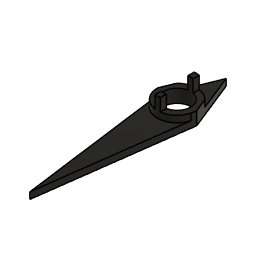
Clock v25 (Autodesk Fusion 360 archive; units mm, degrees)
design "5 lancetta minuti"
Autodesk Fusion 360 part; units mm, degrees
sketch "Schizzo1" plane through (0, 0, 0) normal (0, 0, 1) x (1, 0, 0)
  line L0 (0, -45) -> (6, 0)
  line L1 (6, 0) -> (0, 15)
  line L2 (0, 15) -> (-6, 0)
  line L3 (-6, 0) -> (0, -45)
  line L4 (0, -45) -> (0, 15) construction
  line L5 (6, 0) -> (-6, 0) construction
  circle A0 centre (0, 0) radius 4.15
  circle A1 centre (0, 0) radius 6 construction
  dimension "d1" = 45
  dimension "d2" = 15
  dimension "d3" = 6
  dimension "d12" = 8.3
  dimension "d15" = 12
  constraint vertical L4
  constraint perpendicular L4 L5
  constraint midpoint A0.centre L5
  constraint equal L0 L3
  constraint equal L1 L2
  constraint coincident A0.centre A1.centre
  measures "d1" vertical distance of L0.start L0.end
  measures "d2" vertical distance of L0.end L1.end
  measures "d3" horizontal distance of L0.start L0.end
  measures "d12" diameter of A0
  measures "d15" diameter of A1
extrude "Estrusione1" add sketch "Schizzo1" along normal blind 2
sketch "Schizzo2" plane through (0, 0, 2) normal (0, 0, 1) x (-1, 0, 0)
  line L0 (6, 0) -> (0, 45)
  line L1 (0, 45) -> (-6, 0)
  line L2 (-6, 0) -> (0, -15)
  line L3 (0, -15) -> (6, 0)
  circle A0 centre (0, 0) radius 6
  circle A1 centre (0, 0) radius 4.15
  line L4 (-0.8, 24) -> (0.8, 24)
  line L5 (0.8, 24) -> (0.8, -21)
  line L6 (0.8, -21) -> (-0.8, -21)
  line L7 (-0.8, -21) -> (-0.8, 24)
  circle A2 centre (0, 0) radius 4.15
  circle A3 centre (0, 0) radius 4.15
  line L8 (6, 0) -> (0, 45)
  line L9 (0, 45) -> (-6, 0)
  line L10 (-6, 0) -> (0, -15)
  line L11 (0, -15) -> (6, 0)
  dimension "d6" = 12
  dimension "d7" = 8.3
  dimension "d8" = 0.8
  dimension "d9" = 0.8
  constraint coincident A0.centre A1.centre
  constraint horizontal L4
  constraint vertical L5
  constraint horizontal L6
  constraint vertical L7
  measures "d6" diameter of A0
  measures "d7" diameter of A1
  measures "d8" distance of A0.centre L7
  measures "d9" distance of A0.centre L5
extrude "Estrusione2" add sketch "Schizzo2" along normal blind 5.8 contours A0 A1 L5 L7 A2 A3 | A0 A1 L5 L7 A2 A3
sketch "Schizzo3" plane through (0, 0, 2) normal (0, 0, 1) x (-1, 0, 0)
  line L0 (-0.8, 4.0722) -> (-0.8, 5.9464)
  arc A0 (0.8, 5.9464) -> (-0.8, 5.9464) centre (0, 0) ccw
  line L1 (0.8, 5.9464) -> (0.8, 4.0722)
  arc A1 (0.8, -4.0722) -> (0.8, 4.0722) centre (0, 0) ccw
  line L2 (0.8, -4.0722) -> (0.8, -5.9464)
  arc A2 (-0.8, -5.9464) -> (0.8, -5.9464) centre (0, 0) ccw
  line L3 (-0.8, -5.9464) -> (-0.8, -4.0722)
  arc A3 (-0.8, 4.0722) -> (-0.8, -4.0722) centre (0, 0) ccw
  line L4 (6, 0) -> (0, 45)
  line L5 (0, 45) -> (-6, 0)
  line L6 (-6, 0) -> (0, -15)
  line L7 (0, -15) -> (6, 0)
  circle A4 centre (0, 0) radius 4.15
  circle A5 centre (0, 0) radius 6
  constraint concentric A0 A4
  constraint coincident L3.end A4
  constraint concentric A4 A5
  constraint coincident A2.start A5
extrude "Estrusione3" add sketch "Schizzo3" along normal blind 2 contours L0 L3 A3 L5 L6 A4 A5 | L1 A1 L2 L4 L7 A4 A5

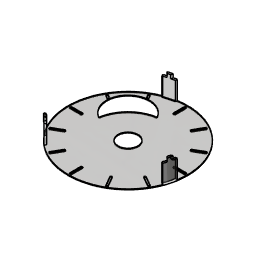
design "10 quadrante"
Autodesk Fusion 360 part; units mm, degrees
sketch "Schizzo1" plane through (0, 0, 0) normal (0, 0, 1) x (1, 0, 0)
  circle A0 centre (0, 0) radius 60
  circle A1 centre (0, 0) radius 10
  circle A2 centre (0, 0) radius 35
  circle A3 centre (-24.0416, 24.0416) radius 21.5
  line L0 (-24.0416, 24.0416) -> (0, 0)
  line L1 (20, 0) -> (2.5, 0)
  dimension "d1" = 120
  dimension "d2" = 20
  dimension "d3" = 70
  dimension "d4" = 43
  dimension "d5" = 135
  dimension "d6" = 34
  constraint coincident A0.centre A1.centre
  constraint concentric A1 A2
  constraint coincident A3.centre L0.start
  measures "d1" diameter of A0
  measures "d2" diameter of A1
  measures "d3" diameter of A2
  measures "d4" diameter of A3
  measures "d5" angle of L0 L1
  measures "d6" distance of A3.centre A0.centre
extrude "Estrusione1" add sketch "Schizzo1" along normal blind 0.8 contours A0 | A2 A3 | A2 A3 picked at (-21.1756, -5.4075) picked at (-19.4046, 19.4046)
sketch "Schizzo2" plane through (0, 0, 0.8) normal (0, 0, 1) x (-1, 0, 0)
  arc A0 (5.3099, -34.5949) -> (34.5949, -5.3099) centre (24.0416, -24.0416) ccw
  arc A1 (5.3099, -34.5949) -> (34.5949, -5.3099) centre (0, 0) ccw
  circle A2 centre (0, 0) radius 10
  circle A3 centre (0, 0) radius 60
  circle A4 centre (0, 0) radius 60
  circle A5 centre (0, 0) radius 58
  circle A6 centre (-57.9555, 15.5291) radius 6
  circle A7 centre (42.4264, 42.4264) radius 6
  circle A8 centre (15.5291, -57.9555) radius 6
  line L0 (15.5291, -57.9555) -> (0, 0) construction
  line L1 (0, 0) -> (-57.9555, 15.5291) construction
  line L2 (0, 0) -> (42.4264, 42.4264) construction
  line L3 (-20, 0) -> (-2.5, 0)
  dimension "d9" = 116
  dimension "d10" = 12
  dimension "d11" = 12
  dimension "d12" = 12
  dimension "d15" = 120
  dimension "d16" = 120
  dimension "d17" = 120
  dimension "d18" = 75
  constraint concentric A1 A4
  constraint concentric A4 A5
  constraint coincident A3 A6.centre
  constraint coincident A4 A7.centre
  constraint coincident A4 A8.centre
  constraint coincident A8.centre L0.start
  constraint coincident A1.centre A2.centre
  constraint coincident A6.centre L1.end
  constraint coincident A7.centre L2.end
  measures "d9" diameter of A5
  measures "d10" diameter of A6
  measures "d11" diameter of A7
  measures "d12" diameter of A8
  measures "d15" angle of L0 L2
  measures "d16" angle of L0 L1
  measures "d17" diameter of A4
  measures "d18" angle of L0 L3
extrude "Estrusione2" add sketch "Schizzo2" along normal blind 18.5 contours A3 A4 A5 A7 | A3 A4 A5 A8 | A3 A4 A5 A6
sketch "Schizzo3" plane through (0, 0, 19.3) normal (0, 0, 1) x (-1, 0, 0)
  arc A0 (9.5764, -57.204) -> (9.6632, -59.2167) centre (15.5291, -57.9555) ccw
  arc A1 (9.6632, -59.2167) -> (21.2398, -56.1148) centre (0, 0) ccw
  arc A2 (21.2398, -56.1148) -> (20.3086, -54.3283) centre (15.5291, -57.9555) ccw
  arc A3 (9.5764, -57.204) -> (20.3086, -54.3283) centre (0, 0) ccw
  circle A4 centre (15.5291, -57.9555) radius 2.5
  dimension "d19" = 5
  constraint concentric A0 A4
  measures "d19" diameter of A4
extrude "Estrusione3" add sketch "Schizzo3" along normal blind 3.5 contours A1 A3 A4
pattern_circular "Serie C1" count 3 over 360 about axis through (0, 0, 1.75) along (0, 0, 1) of "Estrusione3"
sketch "Schizzo4" plane through (0, 0, 0) normal (0, 0, -1) x (1, 0, 0)
  arc A0 (-34.5949, -5.3099) -> (-5.3099, -34.5949) centre (-24.0416, -24.0416) ccw
  arc A1 (-34.5949, -5.3099) -> (-5.3099, -34.5949) centre (0, 0) ccw
  circle A2 centre (0, 0) radius 10
  circle A3 centre (0, 0) radius 60
  line L0 (-58, -0.8) -> (-46, -0.8)
  line L1 (-46, -0.8) -> (-46, 0.8)
  line L2 (-46, 0.8) -> (-58, 0.8)
  line L3 (-58, 0.8) -> (-58, -0.8)
  dimension "d24" = 0.8
  dimension "d25" = 0.8
  dimension "d26" = 58
  dimension "d27" = 12
  constraint horizontal L0
  constraint vertical L1
  constraint horizontal L2
  constraint vertical L3
  measures "d24" distance of A1.centre L0
  measures "d25" distance of A1.centre L2
  measures "d26" distance of A1.centre L3
  measures "d27" distance of L1.end L2.end
extrude "Estrusione4" cut sketch "Schizzo4" against normal blind 0.2 contours L0 L1 L2 L3
pattern_circular "Serie C2" count 12 over 360 about axis through (0, 0, 0) along (0, 0, 1) of "Estrusione4"
sketch "Schizzo5" plane through (0, 0, 0) normal (0, 0, -1) x (1, 0, 0)
  line L0 (0.8, -46) -> (0.8, -58)
  line L1 (0.8, -58) -> (-0.8, -58)
  line L2 (-0.8, -58) -> (-0.8, -46)
  line L3 (-0.8, -46) -> (0.8, -46)
  line L4 (23.6928, -39.4372) -> (29.6928, -49.8295)
  line L5 (29.6928, -49.8295) -> (28.3072, -50.6295)
  line L6 (28.3072, -50.6295) -> (22.3072, -40.2372)
  line L7 (22.3072, -40.2372) -> (23.6928, -39.4372)
  line L8 (40.2372, -22.3072) -> (50.6295, -28.3072)
  line L9 (50.6295, -28.3072) -> (49.8295, -29.6928)
  line L10 (49.8295, -29.6928) -> (39.4372, -23.6928)
  line L11 (39.4372, -23.6928) -> (40.2372, -22.3072)
  line L12 (46, 0.8) -> (58, 0.8)
  line L13 (58, 0.8) -> (58, -0.8)
  line L14 (58, -0.8) -> (46, -0.8)
  line L15 (46, -0.8) -> (46, 0.8)
  line L16 (39.4372, 23.6928) -> (49.8295, 29.6928)
  line L17 (49.8295, 29.6928) -> (50.6295, 28.3072)
  line L18 (50.6295, 28.3072) -> (40.2372, 22.3072)
  line L19 (40.2372, 22.3072) -> (39.4372, 23.6928)
  line L20 (22.3072, 40.2372) -> (28.3072, 50.6295)
  line L21 (28.3072, 50.6295) -> (29.6928, 49.8295)
  line L22 (29.6928, 49.8295) -> (23.6928, 39.4372)
  line L23 (23.6928, 39.4372) -> (22.3072, 40.2372)
  line L24 (-0.8, 46) -> (-0.8, 58)
  line L25 (-0.8, 58) -> (0.8, 58)
  line L26 (0.8, 58) -> (0.8, 46)
  line L27 (0.8, 46) -> (-0.8, 46)
  line L28 (-23.6928, 39.4372) -> (-29.6928, 49.8295)
  line L29 (-29.6928, 49.8295) -> (-28.3072, 50.6295)
  line L30 (-28.3072, 50.6295) -> (-22.3072, 40.2372)
  line L31 (-22.3072, 40.2372) -> (-23.6928, 39.4372)
  line L32 (-40.2372, 22.3072) -> (-50.6295, 28.3072)
  line L33 (-50.6295, 28.3072) -> (-49.8295, 29.6928)
  line L34 (-49.8295, 29.6928) -> (-39.4372, 23.6928)
  line L35 (-39.4372, 23.6928) -> (-40.2372, 22.3072)
  line L36 (-46, -0.8) -> (-58, -0.8)
  line L37 (-58, -0.8) -> (-58, 0.8)
  line L38 (-58, 0.8) -> (-46, 0.8)
  line L39 (-46, 0.8) -> (-46, -0.8)
  line L40 (-45.3242, -27.0917) -> (-49.8295, -29.6928)
  line L41 (-49.8295, -29.6928) -> (-50.6295, -28.3072)
  line L42 (-50.6295, -28.3072) -> (-45.502, -25.3468)
  arc A0 (-34.5949, -5.3099) -> (-45.502, -25.3468) centre (-24.0416, -24.0416) ccw
  arc A1 (-34.5949, -5.3099) -> (-5.3099, -34.5949) centre (0, 0) ccw
  arc A2 (-25.3468, -45.502) -> (-5.3099, -34.5949) centre (-24.0416, -24.0416) ccw
  line L43 (-25.3468, -45.502) -> (-28.3072, -50.6295)
  line L44 (-28.3072, -50.6295) -> (-29.6928, -49.8295)
  line L45 (-29.6928, -49.8295) -> (-27.0917, -45.3242)
  arc A3 (-45.3242, -27.0917) -> (-27.0917, -45.3242) centre (-24.0416, -24.0416) ccw
  circle A4 centre (0, 0) radius 10
  circle A5 centre (0, 0) radius 60
  circle A6 centre (0, 0) radius 35
  circle A7 centre (-24.0416, -24.0416) radius 22.5
  circle A8 centre (-24.0416, -24.0416) radius 21.5
  dimension "d32" = 45
  dimension "d37" = 43
  constraint coincident A1.centre A4.centre
  constraint concentric A3 A7
  constraint concentric A7 A8
  measures "d32" diameter of A7
  measures "d37" diameter of A8
extrude "Estrusione5" add sketch "Schizzo5" along normal up to near side of body 1 contours L40 L42 A7 A8 | L43 L45 A7 A8
sketch "Schizzo7" plane through (0, 0, 0) normal (0, 0, -1) x (1, 0, 0)
  line L0 (-46.2539, -27.6285) -> (-49.8295, -29.6928)
  line L1 (-49.8295, -29.6928) -> (-50.6295, -28.3072)
  line L2 (-50.6295, -28.3072) -> (-46.4645, -25.9026)
  arc A0 (-46.4645, -25.9026) -> (-46.2539, -27.6285) centre (-24.0416, -24.0416) ccw
  line L3 (-25.9026, -46.4645) -> (-28.3072, -50.6295)
  line L4 (-28.3072, -50.6295) -> (-29.6928, -49.8295)
  line L5 (-29.6928, -49.8295) -> (-27.6285, -46.2539)
  arc A1 (-27.6285, -46.2539) -> (-25.9026, -46.4645) centre (-24.0416, -24.0416) ccw
  line L6 (0.8, -46) -> (0.8, -58)
  line L7 (0.8, -58) -> (-0.8, -58)
  line L8 (-0.8, -58) -> (-0.8, -46)
  line L9 (-0.8, -46) -> (0.8, -46)
  line L10 (23.6928, -39.4372) -> (29.6928, -49.8295)
  line L11 (29.6928, -49.8295) -> (28.3072, -50.6295)
  line L12 (28.3072, -50.6295) -> (22.3072, -40.2372)
  line L13 (22.3072, -40.2372) -> (23.6928, -39.4372)
  line L14 (40.2372, -22.3072) -> (50.6295, -28.3072)
  line L15 (50.6295, -28.3072) -> (49.8295, -29.6928)
  line L16 (49.8295, -29.6928) -> (39.4372, -23.6928)
  line L17 (39.4372, -23.6928) -> (40.2372, -22.3072)
  line L18 (46, 0.8) -> (58, 0.8)
  line L19 (58, 0.8) -> (58, -0.8)
  line L20 (58, -0.8) -> (46, -0.8)
  line L21 (46, -0.8) -> (46, 0.8)
  line L22 (39.4372, 23.6928) -> (49.8295, 29.6928)
  line L23 (49.8295, 29.6928) -> (50.6295, 28.3072)
  line L24 (50.6295, 28.3072) -> (40.2372, 22.3072)
  line L25 (40.2372, 22.3072) -> (39.4372, 23.6928)
  line L26 (22.3072, 40.2372) -> (28.3072, 50.6295)
  line L27 (28.3072, 50.6295) -> (29.6928, 49.8295)
  line L28 (29.6928, 49.8295) -> (23.6928, 39.4372)
  line L29 (23.6928, 39.4372) -> (22.3072, 40.2372)
  line L30 (-0.8, 46) -> (-0.8, 58)
  line L31 (-0.8, 58) -> (0.8, 58)
  line L32 (0.8, 58) -> (0.8, 46)
  line L33 (0.8, 46) -> (-0.8, 46)
  line L34 (-23.6928, 39.4372) -> (-29.6928, 49.8295)
  line L35 (-29.6928, 49.8295) -> (-28.3072, 50.6295)
  line L36 (-28.3072, 50.6295) -> (-22.3072, 40.2372)
  line L37 (-22.3072, 40.2372) -> (-23.6928, 39.4372)
  line L38 (-40.2372, 22.3072) -> (-50.6295, 28.3072)
  line L39 (-50.6295, 28.3072) -> (-49.8295, 29.6928)
  line L40 (-49.8295, 29.6928) -> (-39.4372, 23.6928)
  line L41 (-39.4372, 23.6928) -> (-40.2372, 22.3072)
  line L42 (-46, -0.8) -> (-58, -0.8)
  line L43 (-58, -0.8) -> (-58, 0.8)
  line L44 (-58, 0.8) -> (-46, 0.8)
  line L45 (-46, 0.8) -> (-46, -0.8)
  circle A2 centre (0, 0) radius 12.5
  arc A3 (-34.5949, -5.3099) -> (-5.3099, -34.5949) centre (-24.0416, -24.0416) ccw
  arc A4 (-34.5949, -5.3099) -> (-5.3099, -34.5949) centre (0, 0) ccw
  circle A5 centre (0, 0) radius 60
extrude "Estrusione6" cut sketch "Schizzo7" against normal up to surface (0.8 mm away) contours L0 L1 L2 A0 | L3 L4 L5 A1 | L6 L7 L8 L9 | L10 L11 L12 L13 | L14 L15 L16 L17 | L18 L19 L20 L21 | L22 L23 L24 L25 | L26 L27 L28 L29 | L30 L31 L32 L33 | L34 L35 L36 L37 | L38 L39 L40 L41 | L42 L43 L44 L45

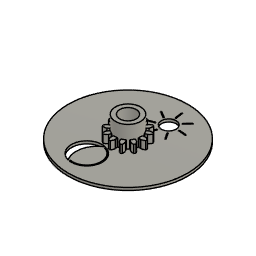
design "9 night and day"
description: Spur Gear; Module: 1.000000; Num Teeth: 12; Pressure Angle: 20.000000; Backlash: 0.00 mm
Autodesk Fusion 360 part; units mm, degrees
sketch "Schizzo1" plane through (0, 0, 0) normal (0, 0, 1) x (1, 0, 0)
  circle A0 centre (0, 0) radius 22.5
  dimension "d1" = 45
  constraint coincident A0.centre origin
  measures "d1" diameter of A0
extrude "Estrusione1" add sketch "Schizzo1" along normal blind 1 makes body 1
sketch "Schizzo1 (2)" plane through (0, 0, 0) normal (0, 0, 1) x (1, 0, 0) in component "Spur Gear (12 teeth)"
  circle A0 centre (0, 0) radius 4.7492
extrude "Estrusione1'" add sketch "Schizzo1 (2)" along normal blind 5 separate body makes body 2 in component "Spur Gear (12 teeth)"
sketch "Schizzo2" plane through (0, 0, 0) normal (0, 0, 1) x (1, 0, 0) in component "Spur Gear (12 teeth)"
  spline S0 degree 5 poles (5.5783, -0.8192) (5.5823, -0.8197) (5.5902, -0.8208) (5.6021, -0.8219) (5.6181, -0.8228) (5.6381, -0.8229) (5.6583, -0.8223) (5.6784, -0.8212) (5.6986, -0.8199) (5.7188, -0.8184) (5.7391, -0.8168) (5.7593, -0.8149) (5.7796, -0.8127) (5.7999, -0.8102) (5.8203, -0.8073) (5.8406, -0.8041) (5.861, -0.8006) (5.8814, -0.7969) (5.9018, -0.793) (5.9222, -0.7888) (5.9426, -0.7845) (5.9631, -0.7799) (5.9835, -0.7752) (6.0039, -0.7702) (6.0244, -0.765) (6.0448, -0.7596) (6.0653, -0.7539) (6.0857, -0.7481) (6.1061, -0.7421) (6.1266, -0.7359) (6.147, -0.7295) (6.1675, -0.7229) (6.1879, -0.7161) (6.2083, -0.7092) (6.2288, -0.7021) (6.2492, -0.6947) (6.2696, -0.6873) (6.29, -0.6796) (6.3104, -0.6717) (6.3308, -0.6637) (6.3512, -0.6555) (6.3715, -0.6472) (6.3919, -0.6387) (6.4122, -0.63) (6.4325, -0.6211) (6.4528, -0.6121) (6.4731, -0.6029) (6.4934, -0.5936) (6.5137, -0.5841) (6.5339, -0.5744) (6.5541, -0.5646) (6.5743, -0.5546) (6.5945, -0.5445) (6.6147, -0.5342) (6.6348, -0.5238) (6.655, -0.5132) (6.6751, -0.5024) (6.6951, -0.4915) (6.7152, -0.4805) (6.7352, -0.4693) (6.7552, -0.4579) (6.7752, -0.4464) (6.7952, -0.4348) (6.8151, -0.423) (6.835, -0.4111) (6.8549, -0.399) (6.8747, -0.3867) (6.8945, -0.3744) (6.9143, -0.3619) (6.9341, -0.3492) (6.9538, -0.3364) (6.9695, -0.3261) (6.9813, -0.3182) (6.9892, -0.313) (6.9931, -0.3103) knots 0 0 0 0 0 0 0.01428571 0.02857143 0.04285714 0.05714286 0.07142857 0.08571429 0.1 0.11428571 0.12857143 0.14285714 0.15714286 0.17142857 0.18571429 0.2 0.21428571 0.22857143 0.24285714 0.25714286 0.27142857 0.28571429 0.3 0.31428571 0.32857143 0.34285714 0.35714286 0.37142857 0.38571429 0.4 0.41428571 0.42857143 0.44285714 0.45714286 0.47142857 0.48571429 0.5 0.51428571 0.52857143 0.54285714 0.55714286 0.57142857 0.58571429 0.6 0.61428571 0.62857143 0.64285714 0.65714286 0.67142857 0.68571429 0.7 0.71428571 0.72857143 0.74285714 0.75714286 0.77142857 0.78571429 0.8 0.81428571 0.82857143 0.84285714 0.85714286 0.87142857 0.88571429 0.9 0.91428571 0.92857143 0.94285714 0.95714286 0.97142857 0.98571429 1 1 1 1 1 1
  spline S1 degree 5 poles (5.5783, 0.8192) (5.5823, 0.8197) (5.5902, 0.8208) (5.6021, 0.8219) (5.6181, 0.8228) (5.6381, 0.8229) (5.6583, 0.8223) (5.6784, 0.8212) (5.6986, 0.8199) (5.7188, 0.8184) (5.7391, 0.8168) (5.7593, 0.8149) (5.7796, 0.8127) (5.7999, 0.8102) (5.8203, 0.8073) (5.8406, 0.8041) (5.861, 0.8006) (5.8814, 0.7969) (5.9018, 0.793) (5.9222, 0.7888) (5.9426, 0.7845) (5.9631, 0.7799) (5.9835, 0.7752) (6.0039, 0.7702) (6.0244, 0.765) (6.0448, 0.7596) (6.0653, 0.7539) (6.0857, 0.7481) (6.1061, 0.7421) (6.1266, 0.7359) (6.147, 0.7295) (6.1675, 0.7229) (6.1879, 0.7161) (6.2083, 0.7092) (6.2288, 0.7021) (6.2492, 0.6947) (6.2696, 0.6873) (6.29, 0.6796) (6.3104, 0.6717) (6.3308, 0.6637) (6.3512, 0.6555) (6.3715, 0.6472) (6.3919, 0.6387) (6.4122, 0.63) (6.4325, 0.6211) (6.4528, 0.6121) (6.4731, 0.6029) (6.4934, 0.5936) (6.5137, 0.5841) (6.5339, 0.5744) (6.5541, 0.5646) (6.5743, 0.5546) (6.5945, 0.5445) (6.6147, 0.5342) (6.6348, 0.5238) (6.655, 0.5132) (6.6751, 0.5024) (6.6951, 0.4915) (6.7152, 0.4805) (6.7352, 0.4693) (6.7552, 0.4579) (6.7752, 0.4464) (6.7952, 0.4348) (6.8151, 0.423) (6.835, 0.4111) (6.8549, 0.399) (6.8747, 0.3867) (6.8945, 0.3744) (6.9143, 0.3619) (6.9341, 0.3492) (6.9538, 0.3364) (6.9695, 0.3261) (6.9813, 0.3182) (6.9892, 0.313) (6.9931, 0.3103) knots 0 0 0 0 0 0 0.01428571 0.02857143 0.04285714 0.05714286 0.07142857 0.08571429 0.1 0.11428571 0.12857143 0.14285714 0.15714286 0.17142857 0.18571429 0.2 0.21428571 0.22857143 0.24285714 0.25714286 0.27142857 0.28571429 0.3 0.31428571 0.32857143 0.34285714 0.35714286 0.37142857 0.38571429 0.4 0.41428571 0.42857143 0.44285714 0.45714286 0.47142857 0.48571429 0.5 0.51428571 0.52857143 0.54285714 0.55714286 0.57142857 0.58571429 0.6 0.61428571 0.62857143 0.64285714 0.65714286 0.67142857 0.68571429 0.7 0.71428571 0.72857143 0.74285714 0.75714286 0.77142857 0.78571429 0.8 0.81428571 0.82857143 0.84285714 0.85714286 0.87142857 0.88571429 0.9 0.91428571 0.92857143 0.94285714 0.95714286 0.97142857 0.98571429 1 1 1 1 1 1
  arc A0 (6.9931, -0.3103) -> (6.9931, 0.3103) centre (0, 0) ccw
  line L0 (4.6889, -0.69) -> (5.5783, -0.8192)
  line L1 (4.6889, 0.69) -> (5.5783, 0.8192)
  line L2 (4.6889, -0.69) -> (4.6889, 0.69)
  point P0 (5.6763, -0.8213)
  point P1 (5.7758, -0.8131)
  point P2 (5.8761, -0.7978)
  point P3 (5.977, -0.7767)
  point P4 (6.0784, -0.7502)
  point P5 (6.1802, -0.7187)
  point P6 (6.2821, -0.6825)
  point P7 (6.3842, -0.6419)
  point P8 (6.4862, -0.5969)
  point P9 (6.5882, -0.5477)
  point P10 (6.6899, -0.4943)
  point P11 (6.7914, -0.437)
  point P12 (6.8925, -0.3756)
  point P13 (5.6763, 0.8213)
  point P14 (5.7758, 0.8131)
  point P15 (5.8761, 0.7978)
  point P16 (5.977, 0.7767)
  point P17 (6.0784, 0.7502)
  point P18 (6.1802, 0.7187)
  point P19 (6.2821, 0.6825)
  point P20 (6.3842, 0.6419)
  point P21 (6.4862, 0.5969)
  point P22 (6.5882, 0.5477)
  point P23 (6.6899, 0.4943)
  point P24 (6.7914, 0.437)
  point P25 (6.8925, 0.3756)
extrude "Estrusione2" add sketch "Schizzo2" along normal blind 5 bodies 2 in component "Spur Gear (12 teeth)"
fillet "Raccordo1" radius 0.1 2 edges at (4.6986, -0.6914, 2.5) (4.6986, 0.6914, 2.5) on bodies 2 in component "Spur Gear (12 teeth)"
pattern_circular "Serie C1" count 12 over 360 about axis through (0, 0, 0) along (0, 0, 1) of "Estrusione2", "Raccordo1" in component "Spur Gear (12 teeth)"
sketch "Schizzo3" plane through (0, 0, 0) normal (0, 0, 1) x (1, 0, 0) in component "Spur Gear (12 teeth)"
  circle A0 centre (0, 0) radius 6 construction
combine "Combina1" operation add target body 1 tool bodies 2
extrude "Estrusione2'" cut 1 faces at (0.3611, -1.5413, 5) along direction (0, 0, -1) blind 1 on bodies 1 bodies 1
sketch "Schizzo2 (2)" plane through (0, 0, 4) normal (0, 0, 1) x (-1, 0, 0)
  arc A0 (-4.4499, 1.6593) -> (-4.6834, 0.788) centre (0, 0) ccw
  arc A1 (-4.7964, 0.7056) -> (-4.6834, 0.788) centre (-4.782, 0.8046) ccw
  line L0 (-4.7964, 0.7056) -> (-5.5783, 0.8192)
  spline S0 degree 3 poles (-6.9931, 0.3103) (-6.7925, 0.4447) (-6.5771, 0.5635) (-6.0115, 0.7938) (-5.7809, 0.814) (-5.6435, 0.8238) (-5.6102, 0.8238) (-5.5783, 0.8192) knots -0.02978 -0.02978 -0.02978 -0.02978 -0.021848 -0.021848 -0.009668 -0.009668 0 0 0 0
  arc A2 (-6.9931, 0.3103) -> (-6.9931, -0.3103) centre (0, 0) ccw
  spline S1 degree 3 poles (-5.5783, -0.8192) (-5.6911, -0.8355) (-5.8671, -0.8005) (-6.0076, -0.7707) (-6.1286, -0.7409) (-6.536, -0.586) (-6.7735, -0.4574) (-6.9931, -0.3103) knots -0.176502 -0.176502 -0.176502 -0.176502 -0.131302 -0.131302 -0.079288 -0.079288 0 0 0 0
  line L1 (-5.5783, -0.8192) -> (-4.7964, -0.7056)
  arc A3 (-4.6834, -0.788) -> (-4.7964, -0.7056) centre (-4.782, -0.8046) ccw
  arc A4 (-4.6834, -0.788) -> (-4.4499, -1.6593) centre (0, 0) ccw
  arc A5 (-4.5066, -1.7871) -> (-4.4499, -1.6593) centre (-4.5436, -1.6942) ccw
  line L2 (-4.5066, -1.7871) -> (-5.2406, -2.0798)
  spline S2 degree 3 poles (-6.2114, -3.2278) (-6.1048, -3.0111) (-5.9777, -2.8005) (-5.603, -2.3183) (-5.4134, -2.1855) (-5.2993, -2.1084) (-5.2705, -2.0917) (-5.2406, -2.0798) knots -0.02978 -0.02978 -0.02978 -0.02978 -0.021848 -0.021848 -0.009668 -0.009668 0 0 0 0
  arc A6 (-6.2114, -3.2278) -> (-5.901, -3.7653) centre (0, 0) ccw
  spline S3 degree 3 poles (-4.4214, -3.4986) (-4.5109, -3.5691) (-4.6808, -3.6268) (-4.8174, -3.6712) (-4.9371, -3.7059) (-5.3674, -3.7755) (-5.6373, -3.7829) (-5.901, -3.7653) knots -0.176502 -0.176502 -0.176502 -0.176502 -0.131302 -0.131302 -0.079288 -0.079288 0 0 0 0
  line L3 (-4.4214, -3.4986) -> (-3.801, -3.0093)
  arc A7 (-3.6619, -3.0241) -> (-3.801, -3.0093) centre (-3.739, -3.0878) ccw
  arc A8 (-3.6619, -3.0241) -> (-3.0241, -3.6619) centre (0, 0) ccw
  arc A9 (-3.0093, -3.801) -> (-3.0241, -3.6619) centre (-3.0878, -3.739) ccw
  line L4 (-3.0093, -3.801) -> (-3.4986, -4.4214)
  spline S4 degree 3 poles (-3.7653, -5.901) (-3.7814, -5.6601) (-3.7766, -5.4142) (-3.6932, -4.8092) (-3.5954, -4.5994) (-3.5352, -4.4756) (-3.5185, -4.4467) (-3.4986, -4.4214) knots -0.02978 -0.02978 -0.02978 -0.02978 -0.021848 -0.021848 -0.009668 -0.009668 0 0 0 0
  arc A10 (-3.7653, -5.901) -> (-3.2278, -6.2114) centre (0, 0) ccw
  spline S5 degree 3 poles (-2.0798, -5.2406) (-2.122, -5.3464) (-2.2403, -5.4813) (-2.3364, -5.5881) (-2.4227, -5.678) (-2.7605, -5.9534) (-2.9906, -6.0947) (-3.2278, -6.2114) knots -0.176502 -0.176502 -0.176502 -0.176502 -0.131302 -0.131302 -0.079288 -0.079288 0 0 0 0
  line L5 (-2.0798, -5.2406) -> (-1.7871, -4.5066)
  arc A11 (-1.6593, -4.4499) -> (-1.7871, -4.5066) centre (-1.6942, -4.5436) ccw
  arc A12 (-1.6593, -4.4499) -> (-0.788, -4.6834) centre (0, 0) ccw
  arc A13 (-0.7056, -4.7964) -> (-0.788, -4.6834) centre (-0.8046, -4.782) ccw
  line L6 (-0.7056, -4.7964) -> (-0.8192, -5.5783)
  spline S6 degree 3 poles (-0.3103, -6.9931) (-0.4447, -6.7925) (-0.5635, -6.5771) (-0.7938, -6.0115) (-0.814, -5.7809) (-0.8238, -5.6435) (-0.8238, -5.6102) (-0.8192, -5.5783) knots -0.02978 -0.02978 -0.02978 -0.02978 -0.021848 -0.021848 -0.009668 -0.009668 0 0 0 0
  arc A14 (-0.3103, -6.9931) -> (0.3103, -6.9931) centre (0, 0) ccw
  spline S7 degree 3 poles (0.8192, -5.5783) (0.8355, -5.6911) (0.8005, -5.8671) (0.7707, -6.0076) (0.7409, -6.1286) (0.586, -6.536) (0.4574, -6.7735) (0.3103, -6.9931) knots -0.176502 -0.176502 -0.176502 -0.176502 -0.131302 -0.131302 -0.079288 -0.079288 0 0 0 0
  line L7 (0.8192, -5.5783) -> (0.7056, -4.7964)
  arc A15 (0.788, -4.6834) -> (0.7056, -4.7964) centre (0.8046, -4.782) ccw
  arc A16 (0.788, -4.6834) -> (1.6593, -4.4499) centre (0, 0) ccw
  arc A17 (1.7871, -4.5066) -> (1.6593, -4.4499) centre (1.6942, -4.5436) ccw
  line L8 (1.7871, -4.5066) -> (2.0798, -5.2406)
  spline S8 degree 3 poles (3.2278, -6.2114) (3.0111, -6.1048) (2.8005, -5.9777) (2.3183, -5.603) (2.1855, -5.4134) (2.1084, -5.2993) (2.0917, -5.2705) (2.0798, -5.2406) knots -0.02978 -0.02978 -0.02978 -0.02978 -0.021848 -0.021848 -0.009668 -0.009668 0 0 0 0
  arc A18 (3.2278, -6.2114) -> (3.7653, -5.901) centre (0, 0) ccw
  spline S9 degree 3 poles (3.4986, -4.4214) (3.5691, -4.5109) (3.6268, -4.6808) (3.6712, -4.8174) (3.7059, -4.9371) (3.7755, -5.3674) (3.7829, -5.6373) (3.7653, -5.901) knots -0.176502 -0.176502 -0.176502 -0.176502 -0.131302 -0.131302 -0.079288 -0.079288 0 0 0 0
  line L9 (3.4986, -4.4214) -> (3.0093, -3.801)
  arc A19 (3.0241, -3.6619) -> (3.0093, -3.801) centre (3.0878, -3.739) ccw
  arc A20 (3.0241, -3.6619) -> (3.6619, -3.0241) centre (0, 0) ccw
  arc A21 (3.801, -3.0093) -> (3.6619, -3.0241) centre (3.739, -3.0878) ccw
  line L10 (3.801, -3.0093) -> (4.4214, -3.4986)
  spline S10 degree 3 poles (5.901, -3.7653) (5.6601, -3.7814) (5.4142, -3.7766) (4.8092, -3.6932) (4.5994, -3.5954) (4.4756, -3.5352) (4.4467, -3.5185) (4.4214, -3.4986) knots -0.02978 -0.02978 -0.02978 -0.02978 -0.021848 -0.021848 -0.009668 -0.009668 0 0 0 0
  arc A22 (5.901, -3.7653) -> (6.2114, -3.2278) centre (0, 0) ccw
  spline S11 degree 3 poles (5.2406, -2.0798) (5.3464, -2.122) (5.4813, -2.2403) (5.5881, -2.3364) (5.678, -2.4227) (5.9534, -2.7605) (6.0947, -2.9906) (6.2114, -3.2278) knots -0.176502 -0.176502 -0.176502 -0.176502 -0.131302 -0.131302 -0.079288 -0.079288 0 0 0 0
  line L11 (5.2406, -2.0798) -> (4.5066, -1.7871)
  arc A23 (4.4499, -1.6593) -> (4.5066, -1.7871) centre (4.5436, -1.6942) ccw
  arc A24 (4.4499, -1.6593) -> (4.6834, -0.788) centre (0, 0) ccw
  arc A25 (4.7964, -0.7056) -> (4.6834, -0.788) centre (4.782, -0.8046) ccw
  line L12 (4.7964, -0.7056) -> (5.5783, -0.8192)
  spline S12 degree 3 poles (6.9931, -0.3103) (6.7925, -0.4447) (6.5771, -0.5635) (6.0115, -0.7938) (5.7809, -0.814) (5.6435, -0.8238) (5.6102, -0.8238) (5.5783, -0.8192) knots -0.02978 -0.02978 -0.02978 -0.02978 -0.021848 -0.021848 -0.009668 -0.009668 0 0 0 0
  arc A26 (6.9931, -0.3103) -> (6.9931, 0.3103) centre (0, 0) ccw
  spline S13 degree 3 poles (5.5783, 0.8192) (5.6911, 0.8355) (5.8671, 0.8005) (6.0076, 0.7707) (6.1286, 0.7409) (6.536, 0.586) (6.7735, 0.4574) (6.9931, 0.3103) knots -0.176502 -0.176502 -0.176502 -0.176502 -0.131302 -0.131302 -0.079288 -0.079288 0 0 0 0
  line L13 (5.5783, 0.8192) -> (4.7964, 0.7056)
  arc A27 (4.6834, 0.788) -> (4.7964, 0.7056) centre (4.782, 0.8046) ccw
  arc A28 (4.6834, 0.788) -> (4.4499, 1.6593) centre (0, 0) ccw
  arc A29 (4.5066, 1.7871) -> (4.4499, 1.6593) centre (4.5436, 1.6942) ccw
  line L14 (4.5066, 1.7871) -> (5.2406, 2.0798)
  spline S14 degree 3 poles (6.2114, 3.2278) (6.1048, 3.0111) (5.9777, 2.8005) (5.603, 2.3183) (5.4134, 2.1855) (5.2993, 2.1084) (5.2705, 2.0917) (5.2406, 2.0798) knots -0.02978 -0.02978 -0.02978 -0.02978 -0.021848 -0.021848 -0.009668 -0.009668 0 0 0 0
  arc A30 (6.2114, 3.2278) -> (5.901, 3.7653) centre (0, 0) ccw
  spline S15 degree 3 poles (4.4214, 3.4986) (4.5109, 3.5691) (4.6808, 3.6268) (4.8174, 3.6712) (4.9371, 3.7059) (5.3674, 3.7755) (5.6373, 3.7829) (5.901, 3.7653) knots -0.176502 -0.176502 -0.176502 -0.176502 -0.131302 -0.131302 -0.079288 -0.079288 0 0 0 0
  line L15 (4.4214, 3.4986) -> (3.801, 3.0093)
  arc A31 (3.6619, 3.0241) -> (3.801, 3.0093) centre (3.739, 3.0878) ccw
  arc A32 (3.6619, 3.0241) -> (3.0241, 3.6619) centre (0, 0) ccw
  arc A33 (3.0093, 3.801) -> (3.0241, 3.6619) centre (3.0878, 3.739) ccw
  line L16 (3.0093, 3.801) -> (3.4986, 4.4214)
  spline S16 degree 3 poles (3.7653, 5.901) (3.7814, 5.6601) (3.7766, 5.4142) (3.6932, 4.8092) (3.5954, 4.5994) (3.5352, 4.4756) (3.5185, 4.4467) (3.4986, 4.4214) knots -0.02978 -0.02978 -0.02978 -0.02978 -0.021848 -0.021848 -0.009668 -0.009668 0 0 0 0
  arc A34 (3.7653, 5.901) -> (3.2278, 6.2114) centre (0, 0) ccw
  spline S17 degree 3 poles (2.0798, 5.2406) (2.122, 5.3464) (2.2403, 5.4813) (2.3364, 5.5881) (2.4227, 5.678) (2.7605, 5.9534) (2.9906, 6.0947) (3.2278, 6.2114) knots -0.176502 -0.176502 -0.176502 -0.176502 -0.131302 -0.131302 -0.079288 -0.079288 0 0 0 0
  line L17 (2.0798, 5.2406) -> (1.7871, 4.5066)
  arc A35 (1.6593, 4.4499) -> (1.7871, 4.5066) centre (1.6942, 4.5436) ccw
  arc A36 (1.6593, 4.4499) -> (0.788, 4.6834) centre (0, 0) ccw
  arc A37 (0.7056, 4.7964) -> (0.788, 4.6834) centre (0.8046, 4.782) ccw
  line L18 (0.7056, 4.7964) -> (0.8192, 5.5783)
  spline S18 degree 3 poles (0.3103, 6.9931) (0.4447, 6.7925) (0.5635, 6.5771) (0.7938, 6.0115) (0.814, 5.7809) (0.8238, 5.6435) (0.8238, 5.6102) (0.8192, 5.5783) knots -0.02978 -0.02978 -0.02978 -0.02978 -0.021848 -0.021848 -0.009668 -0.009668 0 0 0 0
  arc A38 (0.3103, 6.9931) -> (-0.3103, 6.9931) centre (0, 0) ccw
  spline S19 degree 3 poles (-0.8192, 5.5783) (-0.8355, 5.6911) (-0.8005, 5.8671) (-0.7707, 6.0076) (-0.7409, 6.1286) (-0.586, 6.536) (-0.4574, 6.7735) (-0.3103, 6.9931) knots -0.176502 -0.176502 -0.176502 -0.176502 -0.131302 -0.131302 -0.079288 -0.079288 0 0 0 0
  line L19 (-0.8192, 5.5783) -> (-0.7056, 4.7964)
  arc A39 (-0.788, 4.6834) -> (-0.7056, 4.7964) centre (-0.8046, 4.782) ccw
  arc A40 (-0.788, 4.6834) -> (-1.6593, 4.4499) centre (0, 0) ccw
  arc A41 (-1.7871, 4.5066) -> (-1.6593, 4.4499) centre (-1.6942, 4.5436) ccw
  line L20 (-1.7871, 4.5066) -> (-2.0798, 5.2406)
  spline S20 degree 3 poles (-3.2278, 6.2114) (-3.0111, 6.1048) (-2.8005, 5.9777) (-2.3183, 5.603) (-2.1855, 5.4134) (-2.1084, 5.2993) (-2.0917, 5.2705) (-2.0798, 5.2406) knots -0.02978 -0.02978 -0.02978 -0.02978 -0.021848 -0.021848 -0.009668 -0.009668 0 0 0 0
  arc A42 (-3.2278, 6.2114) -> (-3.7653, 5.901) centre (0, 0) ccw
  spline S21 degree 3 poles (-3.4986, 4.4214) (-3.5691, 4.5109) (-3.6268, 4.6808) (-3.6712, 4.8174) (-3.7059, 4.9371) (-3.7755, 5.3674) (-3.7829, 5.6373) (-3.7653, 5.901) knots -0.176502 -0.176502 -0.176502 -0.176502 -0.131302 -0.131302 -0.079288 -0.079288 0 0 0 0
  line L21 (-3.4986, 4.4214) -> (-3.0093, 3.801)
  arc A43 (-3.0241, 3.6619) -> (-3.0093, 3.801) centre (-3.0878, 3.739) ccw
  arc A44 (-3.0241, 3.6619) -> (-3.6619, 3.0241) centre (0, 0) ccw
  arc A45 (-3.801, 3.0093) -> (-3.6619, 3.0241) centre (-3.739, 3.0878) ccw
  line L22 (-3.801, 3.0093) -> (-4.4214, 3.4986)
  spline S22 degree 3 poles (-5.901, 3.7653) (-5.6601, 3.7814) (-5.4142, 3.7766) (-4.8092, 3.6932) (-4.5994, 3.5954) (-4.4756, 3.5352) (-4.4467, 3.5185) (-4.4214, 3.4986) knots -0.02978 -0.02978 -0.02978 -0.02978 -0.021848 -0.021848 -0.009668 -0.009668 0 0 0 0
  arc A46 (-5.901, 3.7653) -> (-6.2114, 3.2278) centre (0, 0) ccw
  spline S23 degree 3 poles (-5.2406, 2.0798) (-5.3464, 2.122) (-5.4813, 2.2403) (-5.5881, 2.3364) (-5.678, 2.4227) (-5.9534, 2.7605) (-6.0947, 2.9906) (-6.2114, 3.2278) knots -0.176502 -0.176502 -0.176502 -0.176502 -0.131302 -0.131302 -0.079288 -0.079288 0 0 0 0
  line L23 (-5.2406, 2.0798) -> (-4.5066, 1.7871)
  arc A47 (-4.4499, 1.6593) -> (-4.5066, 1.7871) centre (-4.5436, 1.6942) ccw
  circle A48 centre (0, 0) radius 4.7492
  circle A49 centre (0, 0) radius 3.1
  dimension "d14" = 9.4984
  dimension "d15" = 6.2
  constraint concentric A0 A48
  constraint concentric A48 A49
  measures "d14" diameter of A48
  measures "d15" diameter of A49
extrude "Estrusione3" add sketch "Schizzo2 (2)" along normal blind 5 contours A0 A4 A8 A12 A16 A20 A24 A28 A32 A36 A40 A44 A48 bodies 1
sketch "Schizzo3 (2)" plane through (0, 0, 0) normal (0, 0, -1) x (1, 0, 0)
  circle A0 centre (0, 0) radius 22.5
  circle A1 centre (3.1767, -12.1691) radius 2.7952
  line L0 (9.7097, -11.8871) -> (6.8258, -12.1397)
  line L1 (6.8258, -12.1397) -> (6.8538, -12.459)
  line L2 (6.8538, -12.459) -> (9.7377, -12.2064)
  line L3 (9.7377, -12.2064) -> (9.7097, -11.8871)
  line L4 (7.2966, -7.0628) -> (7.0295, -6.8856)
  line L5 (7.0295, -6.8856) -> (5.4289, -9.2978)
  line L6 (5.4289, -9.2978) -> (5.696, -9.475)
  line L7 (5.696, -9.475) -> (7.2966, -7.0628)
  line L8 (1.7531, -5.7644) -> (1.4481, -5.8627)
  line L9 (1.4481, -5.8627) -> (2.3361, -8.618)
  line L10 (2.3361, -8.618) -> (2.6412, -8.5197)
  line L11 (2.6412, -8.5197) -> (1.7531, -5.7644)
  line L12 (-2.7183, -9.2888) -> (-2.8316, -9.5887)
  line L13 (-2.8316, -9.5887) -> (-0.1237, -10.6123)
  line L14 (-0.1237, -10.6123) -> (-0.0104, -10.3125)
  line L15 (-0.0104, -10.3125) -> (-2.7183, -9.2888)
  line L16 (-2.7506, -14.9822) -> (-2.5869, -15.2577)
  line L17 (-2.5869, -15.2577) -> (-0.0983, -13.7789)
  line L18 (-0.0983, -13.7789) -> (-0.262, -13.5033)
  line L19 (-0.262, -13.5033) -> (-2.7506, -14.9822)
  line L20 (1.6804, -18.5572) -> (1.998, -18.601)
  line L21 (1.998, -18.601) -> (2.3934, -15.7333)
  line L22 (2.3934, -15.7333) -> (2.0758, -15.6895)
  line L23 (2.0758, -15.6895) -> (1.6804, -18.5572)
  line L24 (7.2383, -17.3219) -> (7.4705, -17.1009)
  line L25 (7.4705, -17.1009) -> (5.4749, -15.0038)
  line L26 (5.4749, -15.0038) -> (5.2427, -15.2247)
  line L27 (5.2427, -15.2247) -> (7.2383, -17.3219)
  circle A2 centre (-2.9782, 12.5602) radius 5.4022
  circle A3 centre (2.2614, 13.876) radius 7.9312
  circle A4 centre (-2.9782, 12.5602) radius 5.8068
  circle A5 centre (2.2614, 13.876) radius 7.4312
  line L28 (-4.3926, 18.1921) -> (-2.9782, 12.5602) construction
  line L29 (-2.9782, 12.5602) -> (-1.5637, 6.9282) construction
  dimension "d19" = 360
  dimension "d56" = -0.5
  constraint perpendicular L0 L1
  constraint parallel L0 L2
  constraint parallel L1 L3
  constraint concentric A2 A4
  constraint coincident A4 L28.start
  constraint coincident A2.centre A4.centre
  constraint coincident A4 L29.end
  constraint parallel L28 L29
  constraint coincident A3 L28.start
  constraint coincident A3 L29.end
  constraint coincident A2 A3.centre
extrude "Estrusione4" cut sketch "Schizzo3 (2)" against normal up to surface (1 mm away) contours A1 | L0 L1 L2 L3 | L4 L5 L6 L7 | L8 L9 L10 L11 | L12 L13 L14 L15 | L16 L17 L18 L19 | L20 L21 L22 L23 | L24 L25 L26 L27 | A2 A4 A5 | A2 A3 | A2 A3 A4 bodies 1
component "Spur Gear (12 teeth)" placed x (1, 0, 0) y (0, 1, 0) z (0, 0, 1) at (0, 0, 0)
